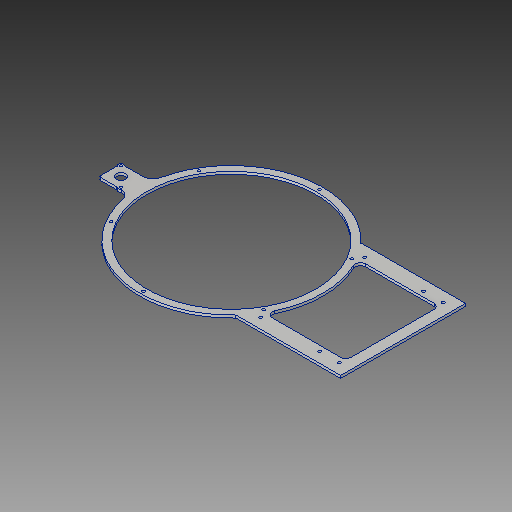
# Autodesk Inventor part: Turret Support 2
Saved by Autodesk Inventor 2019.4 (Build 234330000, 330)
## iProperties
Created: 2020-01-19
Part Number: Turret Support 2
Material: Aluminum 6061
Document SubType Name: Modeling
Designer: Mark
Mass: 421.62 g
Surface Area: 801.814 cm^2
Volume: 156.156 cm^3
Density: 2.7 g/cm^3
Appearance: Aluminum - Flat
Author: Mark
Autodesk Inventor part; units mm, degrees
ref_plane "YZ Plane" through (0, 0, 0) normal (1, 0, 0) x (0, 1, 0)
ref_plane "XZ Plane" through (0, 0, 0) normal (0, 1, 0) x (-1, 0, 0)
ref_plane "XY Plane" through (0, 0, 0) normal (0, 0, 1) x (1, 0, 0)
sketch "Sketch1" plane through (0, 0, 0) normal (0, 1, 0) x (-1, 0, 0)
  circle A0 centre (0, 0) radius 175
  circle A1 centre (0, 0) radius 161.5
  dimension "d0" = 350
  dimension "d1" = 323
  constraints: 2 centre point, 2 coincident
  measures "d0" diameter of A0
  measures "d1" diameter of A1
extrude "Extrusion1" add sketch "Sketch1" along normal blind 5
sketch "Sketch2" plane through (0, 5, 0) normal (0, 1, 0) x (1, 0, 0)
  circle A0 centre (0, 0) radius 175 projected
  line L0 (-128.0332, -119.3) -> (128.0332, -119.3)
  line L1 (128.0332, -119.3) -> (128.0332, 119.3)
  line L2 (128.0332, 119.3) -> (-128.0332, 119.3)
  line L3 (-128.0332, 119.3) -> (-128.0332, -119.3)
  line L4 (-128.0332, -119.3) -> (128.0332, 119.3) construction
  line L5 (128.0332, -119.3) -> (-128.0332, 119.3) construction
  line L6 (128.0332, -119.3) -> (328.0332, -119.3)
  line L7 (328.0332, -119.3) -> (328.0332, 119.3)
  line L8 (328.0332, 119.3) -> (128.0332, 119.3)
  line L9 (128.0332, 119.3) -> (128.0332, -119.3)
  dimension "d4" = 238.6
  dimension "d5" = 200
  dimension "d6" = 238.6
  constraints: 20 end point, 4 parallel, 2 horizontal, 2 midpoint, 2 perpendicular, 1 point on circle
  measures "d4" distance of L0.end L1.end
  measures "d5" distance of L8.end L7.end
  measures "d6" distance of L7.end L6.end
extrude "Extrusion2" add sketch "Sketch2" against normal blind 5 contours A0 L1 | A0 L8 L7 L6
sketch "Sketch3" plane through (0, 5, 0) normal (0, 1, 0) x (1, 0, 0)
  circle A0 centre (0, 0) radius 161.5
  line L0 (328.0332, 119.3) -> (328.0332, -119.3) projected
  line L1 (328.0332, 89.3) -> (168.0332, 89.3)
  line L2 (168.0332, -89.3) -> (328.0332, -89.3)
  line L3 (328.0332, -89.3) -> (328.0332, 89.3)
  line L4 (328.0332, 119.3) -> (128.0332, 119.3) projected
  line L5 (128.0332, -119.3) -> (328.0332, -119.3) projected
  arc A1 (128.0332, 119.3) -> (128.0332, -119.3) centre (0, 0) ccw projected
  arc A2 (150.5009, -89.3) -> (150.5009, 89.3) centre (0, 0) ccw
  line L6 (168.0332, 89.3) -> (150.5009, 89.3)
  line L7 (168.0332, -89.3) -> (150.5009, -89.3)
  dimension "d9" = 323
  dimension "d10" = 30
  dimension "d11" = 30
  dimension "d12" = 160
  dimension "d16" = 175
  constraints: 10 end point, 2 centre point, 2 horizontal, 2 point on circle, 1 coincident, 1 collinear, 1 concentric, 1 parallel, 1 point on line
  measures "d9" diameter of A0
  measures "d10" distance between parallel lines of L4 L1
  measures "d11" distance between parallel lines of L5 L2
  measures "d12" distance of L2.start L2.end
  measures "d16" radius of A2
extrude "Extrusion3" cut sketch "Sketch3" against normal blind 5 contours A0 | L0 L2 L7 A2 L6 L1
fillet "Fillet1" radius 10 2 edges at (150.5009, 2.5, -89.3) (150.5009, 2.5, 89.3)
sketch "Sketch4" plane through (0, 5, 0) normal (0, 1, 0) x (1, 0, 0)
  line L0 (328.0332, -119.3) -> (328.0332, -89.3) projected
  line L1 (328.0332, -89.3) -> (308.0332, -89.3)
  line L2 (308.0332, -89.3) -> (308.0332, 110.7)
  line L3 (308.0332, 110.7) -> (328.0332, 110.7)
  line L4 (328.0332, 110.7) -> (328.0332, -89.3)
  point P0 (0, 0)
  dimension "d17" = 20
  dimension "d18" = 200
  constraints: 8 end point, 2 parallel, 1 horizontal, 1 perpendicular
  measures "d17" distance of L2.end L3.end
  measures "d18" distance of L1.end L2.end
extrude "Extrusion4" add sketch "Sketch4" against normal blind 5
fillet "Fillet2" radius 10 2 edges at (308.0332, 2.5, 89.3) (308.0332, 2.5, -89.3)
sketch "Sketch5" plane through (0, 5, 0) normal (0, 1, 0) x (1, 0, 0)
  circle A0 centre (305.3762, 99.3) radius 2.75
  circle A1 centre (155.3762, 99.3) radius 2.75
  circle A2 centre (305.3762, -99.3) radius 2.75
  circle A3 centre (155.3762, -99.3) radius 2.75
  line L0 (128.0332, -119.3) -> (328.0332, -119.3) projected
  line L1 (328.0332, 119.3) -> (128.0332, 119.3) projected
  line L2 (328.0332, -119.3) -> (328.0332, 119.3) projected
  circle A4 centre (267.8762, -99.3) radius 2.75
  circle A5 centre (267.7762, 99.3) radius 2.75
  point P0 (0, 0)
  dimension "d22" = 5.5
  dimension "d23" = 5.5
  dimension "d24" = 5.5
  dimension "d25" = 5.5
  dimension "d26" = 150
  dimension "d27" = 20
  dimension "d28" = 20
  dimension "d29" = 20
  dimension "d30" = 20
  dimension "d31" = 150
  dimension "d32" = 22.657
  dimension "d33" = 22.657
  dimension "d63" = 5.5
  dimension "d64" = 5.5
  dimension "d65" = 20
  dimension "d66" = 20
  dimension "d67" = 37.6
  dimension "d68" = 37.5
  constraints: 6 centre point
  measures "d22" diameter of A0
  measures "d23" diameter of A1
  measures "d24" diameter of A2
  measures "d25" diameter of A3
  measures "d26" distance of A2.centre A3.centre
  measures "d27" distance from line of L0 A2.centre
  measures "d28" distance from line of L0 A3.centre
  measures "d29" distance from line of L1 A0.centre
  measures "d30" distance from line of L1 A1.centre
  measures "d31" distance of A0.centre A1.centre
  measures "d32" distance from line of A0.centre L2
  measures "d33" distance from line of L2 A2.centre
  measures "d63" diameter of A4
  measures "d64" diameter of A5
  measures "d65" distance from line of L0 A4.centre
  measures "d66" distance from line of L1 A5.centre
  measures "d67" distance of A0.centre A5.centre
  measures "d68" distance of A2.centre A4.centre
extrude "Extrusion5" cut sketch "Sketch5" against normal blind 10
sketch "Sketch6" plane through (0, 5, 0) normal (0, 1, 0) x (1, 0, 0)
  circle A0 centre (0, 0) radius 168.25 construction
  line L0 (0, 0) -> (0, -168.25) construction
  line L1 (0, 0) -> (168.25, 0) construction
  circle A1 centre (0, -168.25) radius 2.75
  circle A2 centre (145.7088, -84.125) radius 2.75
  circle A3 centre (145.7088, 84.125) radius 2.75
  circle A4 centre (0, 168.25) radius 2.75
  circle A5 centre (-145.7088, 84.125) radius 2.75
  circle A6 centre (-145.7088, -84.125) radius 2.75
  dimension "d36" = 336.5
  dimension "d37" = 90
  dimension "d38" = 5.5
  dimension "d41" = 360
  constraints: 6 centre point, 4 end point, 2 coincident, 1 horizontal, 1 perpendicular, 1 vertical alignment, 15 other
  measures "d37" angle of L0 L1
  measures "d38" diameter of A1
extrude "Extrusion6" cut sketch "Sketch6" against normal blind 10
sketch "Sketch7" plane through (0, 5, 0) normal (0, 1, 0) x (1, 0, 0)
  line L0 (-173.7354, 21) -> (-232, 21)
  line L1 (-232, 21) -> (-232, -21)
  line L2 (-232, -21) -> (-173.7354, -21)
  arc A0 (128.0332, 119.3) -> (128.0332, -119.3) centre (0, 0) ccw projected
  circle A1 centre (-211, 0) radius 9.5
  dimension "d45" = 211
  dimension "d46" = 21
  dimension "d47" = 42
  dimension "d48" = 21
  dimension "d49" = 19
  constraints: 6 end point, 2 perpendicular, 2 point on circle, 1 centre point, 1 horizontal, 1 parallel
  measures "d45" distance of point (0, 0) A1.centre
  measures "d46" distance from line of L1 A1.centre
  measures "d47" distance of L0.end L1.end
  measures "d48" distance from line of L0 A1.centre
  measures "d49" diameter of A1
extrude "Extrusion7" add sketch "Sketch7" against normal up to surface (5 mm away)
fillet "Fillet3" radius 20 2 edges at (-173.7354, 2.5, 21) (-173.7354, 2.5, -21)
fillet "Fillet4" radius 2 2 edges at (-232, 2.5, 21) (-232, 2.5, -21)
sketch "Sketch9" plane through (0, 5, 0) normal (0, 1, 0) x (1, 0, 0)
  circle A0 centre (-193.0395, -17.9605) radius 2.5 projected
  circle A1 centre (-193.0395, -17.9605) radius 5
  circle A2 centre (-228.9605, 17.9605) radius 2.5 projected
  circle A3 centre (-228.9605, 17.9605) radius 5
  point P0 (0, 0)
  dimension "d58" = 10
  dimension "d59" = 10
  constraints: 2 centre point, 2 coincident
  measures "d58" diameter of A1
  measures "d59" diameter of A3
extrude "Extrusion9" add sketch "Sketch9" against normal up to surface (5 mm away)
fillet "Fillet5" radius 5 2 edges at (-197.0096, 2.5, 21) (-224.9904, 2.5, -21)
sketch "Sketch10" plane through (0, 5, 0) normal (0, 1, 0) x (1, 0, 0)
  circle A0 centre (-228.9605, 17.9605) radius 2.0193 projected
  circle A1 centre (-193.0395, -17.9605) radius 2.0193 projected
  circle A2 centre (-228.9605, 17.9605) radius 2.5
  circle A3 centre (-193.0395, -17.9605) radius 2.5
  point P0 (0, 0)
  dimension "d69" = 5
  dimension "d70" = 5
  constraints: 2 centre point, 2 coincident
  measures "d69" diameter of A2
  measures "d70" diameter of A3
extrude "Extrusion10" cut sketch "Sketch10" against normal through all contours A0 | A1 | A2 | A3
equation "\"d26\" = d31"
equation "\"d27\" = d30"
equation "\"d28\" = d30"
equation "\"d29\" = d30"
equation "\"d33\" = d32"
equation "\"d48\" = d46"
body "Solid1"
